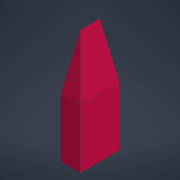
# Autodesk Inventor part: 110033226_ipt_40_背流拱橋裝飾
Saved by Autodesk Inventor 2022 (Build 260153000, 153)
## iProperties
Created: 2022-06-26
Part Number: 110033226_ipt_40_背流拱橋裝飾
Material: 一般
Document SubType Name: Modeling
Designer: User
Density: 1 g/cm^3
Appearance: 預設
Author: User
Autodesk Inventor part; units mm, degrees
ref_plane "YZ Plane" through (0, 0, 0) normal (1, 0, 0) x (0, 1, 0)
ref_plane "XZ Plane" through (0, 0, 0) normal (0, 1, 0) x (-1, 0, 0)
ref_plane "XY Plane" through (0, 0, 0) normal (0, 0, 1) x (1, 0, 0)
sketch "草圖1" plane through (0, 0, 0) normal (0, 1, 0) x (-1, 0, 0)
  line L0 (2.5, 5) -> (-2.5, 5)
  line L1 (-2.5, 5) -> (-2.5, -5)
  line L2 (-2.5, -5) -> (2.5, -5)
  line L3 (2.5, -5) -> (2.5, 5)
  circle A0 centre (0, 2.5) radius 1.7
  point P0 (0, 0)
  point P1 (0, -5)
  point P2 (2.5, 0)
  dimension "d0" = 5
  dimension "d1" = 10
  dimension "d2" = 3.4
  dimension "d3" = 2.5
  dimension "d4" = 2.5
  constraints: 8 end point, 2 midpoint, 2 parallel, 1 centre point, 1 horizontal, 1 horizontal alignment, 1 perpendicular, 1 vertical alignment
  measures "d0" distance of L2.end L1.end
  measures "d1" distance of L1.end L0.end
  measures "d2" diameter of A0
  measures "d3" distance from line of A0.centre L3
  measures "d4" distance from line of L0 A0.centre
extrude "擠出1" add sketch "草圖1" along normal blind 15 contours L3 L2 L1 L0 | A0
extrude "擠出2" cut sketch "草圖1" along normal blind 1.5 contours A0
pattern_linear "矩形陣列1" count 2 spacing 5 along (0, 0, -1) of "擠出2"
sketch "草圖3" plane through (0, 15, 0) normal (0, 1, 0) x (1, 0, 0)
  line L0 (2.5, -5) -> (2.5, 5) projected
  line L1 (2.5, 5) -> (-2.5, 5) projected
  line L2 (-2.5, 5) -> (-2.5, -5) projected
  line L3 (-2.5, -5) -> (2.5, -5) projected
  point P0 (0, 0)
extrude "擠出4" add sketch "草圖3" along normal blind 20 draft -10
